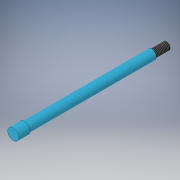
# Autodesk Inventor part: A
Saved by Autodesk Inventor 2017 (Build 210142000, 142)
## iProperties
Part Number: A
Material: 一般
Document SubType Name: Modeling
Designer: user
Density: 1 g/cm^3
Appearance: 青綠色
Author: user
Autodesk Inventor part; units mm, degrees
ref_plane "YZ Plane" through (0, 0, 0) normal (1, 0, 0) x (0, 1, 0)
ref_plane "XZ Plane" through (0, 0, 0) normal (0, 1, 0) x (-1, 0, 0)
ref_plane "XY Plane" through (0, 0, 0) normal (0, 0, 1) x (1, 0, 0)
sketch "草圖1" plane through (0, 0, 0) normal (1, 0, 0) x (0, 1, 0)
  line L0 (0, 0) -> (2.5, 0)
  line L1 (2.5, 0) -> (2.5, 68)
  line L2 (2.5, 68) -> (0, 68)
  line L3 (0, 68) -> (0, 0)
  line L4 (0, 0) -> (2, 0)
  line L5 (2, 0) -> (2, -8)
  line L6 (2, -8) -> (0, -8)
  line L7 (0, -8) -> (0, 0)
  line L8 (0, 68) -> (3, 68)
  line L9 (3, 68) -> (3, 74)
  line L10 (3, 74) -> (0, 74)
  line L11 (0, 74) -> (0, 68)
  dimension "d1" = 6
  dimension "d2" = 3
  dimension "d3" = 2.5
  dimension "d4" = 8
  dimension "d5" = 2
  dimension "d6" = 82
  constraints: 24 end point, 6 parallel, 3 horizontal, 3 perpendicular
  measures "d1" distance of L8.end L9.end
  measures "d2" distance of L9.end L10.end
  measures "d3" distance between parallel lines of L3 L1
  measures "d4" distance of L4.end L5.end
  measures "d5" distance between parallel lines of L7 L5
  measures "d6" distance between parallel lines of L6 L10
revolve "迴轉1" add sketch "草圖1" angle 360 about axis through (0, 0, 68) along (0, 0, -1)
thread "螺紋3" size "M4x0.7" class "6g" standard "ANSI Metric M Profile" full length
